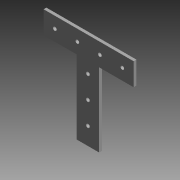
# Autodesk Inventor part: Angle attach bracket
Saved by Autodesk Inventor 2014 (Build 180170000, 170)
## iProperties
Created: 2014-01-19
Part Number: Angle attach bracket
Material: Generic
Document SubType Name: Sheet Metal
Designer: intern
Density: 1 g/cm^3
Sheet Metal Rule: Default
Appearance: Default
Author: intern
Autodesk Inventor part; units mm, degrees
ref_plane "YZ Plane" through (0, 0, 0) normal (1, 0, 0) x (0, 1, 0)
ref_plane "XZ Plane" through (0, 0, 0) normal (0, 1, 0) x (-1, 0, 0)
ref_plane "XY Plane" through (0, 0, 0) normal (0, 0, 1) x (1, 0, 0)
sketch "Sketch1" plane through (0, 0, 0) normal (0, 0, 1) x (1, 0, 0)
  line L0 (0, -83.185) -> (12.6238, -83.185)
  line L1 (12.6238, -83.185) -> (12.6238, -65.5687)
  arc A0 (12.6238, -61.4313) -> (12.6238, -65.5687) centre (12.7, -63.5) ccw
  line L2 (12.6238, -61.4313) -> (12.6238, -40.1687)
  arc A1 (12.6238, -36.0313) -> (12.6238, -40.1687) centre (12.7, -38.1) ccw
  line L3 (12.6238, -36.0313) -> (12.6238, -14.7687)
  arc A2 (12.6238, -10.6313) -> (12.6238, -14.7687) centre (12.7, -12.7) ccw
  line L4 (12.6238, -10.6313) -> (12.6238, 0)
  line L5 (0, 0) -> (12.6238, 0)
  line L6 (0, 0) -> (0, -83.185)
  line L7 (12.7762, -83.185) -> (25.4, -83.185)
  line L8 (25.4, 0) -> (25.4, -83.185)
  line L9 (12.7762, 0) -> (25.4, 0)
  line L10 (12.7762, -10.6313) -> (12.7762, 0)
  arc A3 (12.7762, -14.7687) -> (12.7762, -10.6313) centre (12.7, -12.7) ccw
  line L11 (12.7762, -36.0313) -> (12.7762, -14.7687)
  arc A4 (12.7762, -40.1687) -> (12.7762, -36.0313) centre (12.7, -38.1) ccw
  line L12 (12.7762, -61.4313) -> (12.7762, -40.1687)
  arc A5 (12.7762, -65.5687) -> (12.7762, -61.4313) centre (12.7, -63.5) ccw
  line L13 (12.7762, -83.185) -> (12.7762, -65.5687)
  line L14 (216.6911, 0) -> (216.6911, 12.6238)
  line L15 (216.6911, 12.6238) -> (206.0725, 12.6238)
  arc A6 (201.9097, 12.6238) -> (206.0725, 12.6238) centre (203.9911, 12.7) ccw
  line L16 (201.9097, 12.6238) -> (180.6725, 12.6238)
  arc A7 (176.5097, 12.6238) -> (180.6725, 12.6238) centre (178.5911, 12.7) ccw
  line L17 (176.5097, 12.6238) -> (155.2725, 12.6238)
  arc A8 (151.1097, 12.6238) -> (155.2725, 12.6238) centre (153.1911, 12.7) ccw
  line L18 (151.1097, 12.6238) -> (129.8725, 12.6238)
  arc A9 (125.7097, 12.6238) -> (129.8725, 12.6238) centre (127.7911, 12.7) ccw
  line L19 (125.7097, 12.6238) -> (104.4725, 12.6238)
  arc A10 (100.3097, 12.6238) -> (104.4725, 12.6238) centre (102.3911, 12.7) ccw
  line L20 (100.3097, 12.6238) -> (79.0725, 12.6238)
  arc A11 (74.9097, 12.6238) -> (79.0725, 12.6238) centre (76.9911, 12.7) ccw
  line L21 (74.9097, 12.6238) -> (53.6725, 12.6238)
  arc A12 (49.5097, 12.6238) -> (53.6725, 12.6238) centre (51.5911, 12.7) ccw
  line L22 (49.5097, 12.6238) -> (28.2725, 12.6238)
  arc A13 (24.1097, 12.6238) -> (28.2725, 12.6238) centre (26.1911, 12.7) ccw
  line L23 (24.1097, 12.6238) -> (2.8725, 12.6238)
  arc A14 (-1.2903, 12.6238) -> (2.8725, 12.6238) centre (0.7911, 12.7) ccw
  line L24 (-1.2903, 12.6238) -> (-22.5275, 12.6238)
  arc A15 (-26.6903, 12.6238) -> (-22.5275, 12.6238) centre (-24.6089, 12.7) ccw
  line L25 (-26.6903, 12.6238) -> (-47.9275, 12.6238)
  arc A16 (-52.0903, 12.6238) -> (-47.9275, 12.6238) centre (-50.0089, 12.7) ccw
  line L26 (-52.0903, 12.6238) -> (-73.3275, 12.6238)
  arc A17 (-77.4903, 12.6238) -> (-73.3275, 12.6238) centre (-75.4089, 12.7) ccw
  line L27 (-77.4903, 12.6238) -> (-98.7275, 12.6238)
  arc A18 (-102.8903, 12.6238) -> (-98.7275, 12.6238) centre (-100.8089, 12.7) ccw
  line L28 (-102.8903, 12.6238) -> (-124.1275, 12.6238)
  arc A19 (-128.2903, 12.6238) -> (-124.1275, 12.6238) centre (-126.2089, 12.7) ccw
  line L29 (-128.2903, 12.6238) -> (-149.5275, 12.6238)
  arc A20 (-153.6903, 12.6238) -> (-149.5275, 12.6238) centre (-151.6089, 12.7) ccw
  line L30 (-153.6903, 12.6238) -> (-174.9275, 12.6238)
  arc A21 (-179.0903, 12.6238) -> (-174.9275, 12.6238) centre (-177.0089, 12.7) ccw
  line L31 (-179.0903, 12.6238) -> (-200.3275, 12.6238)
  arc A22 (-204.4903, 12.6238) -> (-200.3275, 12.6238) centre (-202.4089, 12.7) ccw
  line L32 (-204.4903, 12.6238) -> (-225.7275, 12.6238)
  arc A23 (-229.8903, 12.6238) -> (-225.7275, 12.6238) centre (-227.8089, 12.7) ccw
  line L33 (-229.8903, 12.6238) -> (-251.1275, 12.6238)
  arc A24 (-255.2903, 12.6238) -> (-251.1275, 12.6238) centre (-253.2089, 12.7) ccw
  line L34 (-255.2903, 12.6238) -> (-276.5275, 12.6238)
  arc A25 (-280.6903, 12.6238) -> (-276.5275, 12.6238) centre (-278.6089, 12.7) ccw
  line L35 (-280.6903, 12.6238) -> (-301.9275, 12.6238)
  arc A26 (-306.0903, 12.6238) -> (-301.9275, 12.6238) centre (-304.0089, 12.7) ccw
  line L36 (-306.0903, 12.6238) -> (-327.3275, 12.6238)
  arc A27 (-331.4903, 12.6238) -> (-327.3275, 12.6238) centre (-329.4089, 12.7) ccw
  line L37 (-331.4903, 12.6238) -> (-352.7275, 12.6238)
  arc A28 (-356.8903, 12.6238) -> (-352.7275, 12.6238) centre (-354.8089, 12.7) ccw
  line L38 (-356.8903, 12.6238) -> (-378.1275, 12.6238)
  arc A29 (-382.2903, 12.6238) -> (-378.1275, 12.6238) centre (-380.2089, 12.7) ccw
  line L39 (-382.2903, 12.6238) -> (-403.5275, 12.6238)
  arc A30 (-407.6903, 12.6238) -> (-403.5275, 12.6238) centre (-405.6089, 12.7) ccw
  line L40 (-407.6903, 12.6238) -> (-418.3089, 12.6238)
  line L41 (-418.3089, 12.6238) -> (-418.3089, 0)
  line L42 (-418.3089, 0) -> (216.6911, 0)
  line L43 (216.6911, 12.7762) -> (216.6911, 25.4)
  line L44 (-418.3089, 25.4) -> (216.6911, 25.4)
  line L45 (-418.3089, 25.4) -> (-418.3089, 12.7762)
  line L46 (-418.3089, 12.7762) -> (-407.6903, 12.7762)
  arc A31 (-403.5275, 12.7762) -> (-407.6903, 12.7762) centre (-405.6089, 12.7) ccw
  line L47 (-403.5275, 12.7762) -> (-382.2903, 12.7762)
  arc A32 (-378.1275, 12.7762) -> (-382.2903, 12.7762) centre (-380.2089, 12.7) ccw
  line L48 (-378.1275, 12.7762) -> (-356.8903, 12.7762)
  arc A33 (-352.7275, 12.7762) -> (-356.8903, 12.7762) centre (-354.8089, 12.7) ccw
  line L49 (-352.7275, 12.7762) -> (-331.4903, 12.7762)
  arc A34 (-327.3275, 12.7762) -> (-331.4903, 12.7762) centre (-329.4089, 12.7) ccw
  line L50 (-327.3275, 12.7762) -> (-306.0903, 12.7762)
  arc A35 (-301.9275, 12.7762) -> (-306.0903, 12.7762) centre (-304.0089, 12.7) ccw
  line L51 (-301.9275, 12.7762) -> (-280.6903, 12.7762)
  arc A36 (-276.5275, 12.7762) -> (-280.6903, 12.7762) centre (-278.6089, 12.7) ccw
  line L52 (-276.5275, 12.7762) -> (-255.2903, 12.7762)
  arc A37 (-251.1275, 12.7762) -> (-255.2903, 12.7762) centre (-253.2089, 12.7) ccw
  line L53 (-251.1275, 12.7762) -> (-229.8903, 12.7762)
  arc A38 (-225.7275, 12.7762) -> (-229.8903, 12.7762) centre (-227.8089, 12.7) ccw
  line L54 (-225.7275, 12.7762) -> (-204.4903, 12.7762)
  arc A39 (-200.3275, 12.7762) -> (-204.4903, 12.7762) centre (-202.4089, 12.7) ccw
  line L55 (-200.3275, 12.7762) -> (-179.0903, 12.7762)
  arc A40 (-174.9275, 12.7762) -> (-179.0903, 12.7762) centre (-177.0089, 12.7) ccw
  line L56 (-174.9275, 12.7762) -> (-153.6903, 12.7762)
  arc A41 (-149.5275, 12.7762) -> (-153.6903, 12.7762) centre (-151.6089, 12.7) ccw
  line L57 (-149.5275, 12.7762) -> (-128.2903, 12.7762)
  arc A42 (-124.1275, 12.7762) -> (-128.2903, 12.7762) centre (-126.2089, 12.7) ccw
  line L58 (-124.1275, 12.7762) -> (-102.8903, 12.7762)
  arc A43 (-98.7275, 12.7762) -> (-102.8903, 12.7762) centre (-100.8089, 12.7) ccw
  line L59 (-98.7275, 12.7762) -> (-77.4903, 12.7762)
  arc A44 (-73.3275, 12.7762) -> (-77.4903, 12.7762) centre (-75.4089, 12.7) ccw
  line L60 (-73.3275, 12.7762) -> (-52.0903, 12.7762)
  arc A45 (-47.9275, 12.7762) -> (-52.0903, 12.7762) centre (-50.0089, 12.7) ccw
  line L61 (-47.9275, 12.7762) -> (-26.6903, 12.7762)
  arc A46 (-22.5275, 12.7762) -> (-26.6903, 12.7762) centre (-24.6089, 12.7) ccw
  line L62 (-22.5275, 12.7762) -> (-1.2903, 12.7762)
  arc A47 (2.8725, 12.7762) -> (-1.2903, 12.7762) centre (0.7911, 12.7) ccw
  line L63 (2.8725, 12.7762) -> (24.1097, 12.7762)
  arc A48 (28.2725, 12.7762) -> (24.1097, 12.7762) centre (26.1911, 12.7) ccw
  line L64 (28.2725, 12.7762) -> (49.5097, 12.7762)
  arc A49 (53.6725, 12.7762) -> (49.5097, 12.7762) centre (51.5911, 12.7) ccw
  line L65 (53.6725, 12.7762) -> (74.9097, 12.7762)
  arc A50 (79.0725, 12.7762) -> (74.9097, 12.7762) centre (76.9911, 12.7) ccw
  line L66 (79.0725, 12.7762) -> (100.3097, 12.7762)
  arc A51 (104.4725, 12.7762) -> (100.3097, 12.7762) centre (102.3911, 12.7) ccw
  line L67 (104.4725, 12.7762) -> (125.7097, 12.7762)
  arc A52 (129.8725, 12.7762) -> (125.7097, 12.7762) centre (127.7911, 12.7) ccw
  line L68 (129.8725, 12.7762) -> (151.1097, 12.7762)
  arc A53 (155.2725, 12.7762) -> (151.1097, 12.7762) centre (153.1911, 12.7) ccw
  line L69 (155.2725, 12.7762) -> (176.5097, 12.7762)
  arc A54 (180.6725, 12.7762) -> (176.5097, 12.7762) centre (178.5911, 12.7) ccw
  line L70 (180.6725, 12.7762) -> (201.9097, 12.7762)
  arc A55 (206.0725, 12.7762) -> (201.9097, 12.7762) centre (203.9911, 12.7) ccw
  line L71 (206.0725, 12.7762) -> (216.6911, 12.7762)
  line L72 (-37.3089, 25.4) -> (64.2911, 25.4)
  line L73 (64.2911, 25.4) -> (64.2911, 0)
  line L74 (64.2911, 0) -> (-37.3089, 0)
  line L75 (-37.3089, 0) -> (-37.3089, 25.4)
  line L76 (0, 0) -> (25.4, 0)
  line L77 (25.4, 0) -> (25.4, -83.185)
  line L78 (25.4, -83.185) -> (0, -83.185)
  line L79 (0, -83.185) -> (0, 0)
  circle A56 centre (-24.6089, 12.7) radius 2.0828
  circle A57 centre (0.7911, 12.7) radius 2.0828
  circle A58 centre (26.1911, 12.7) radius 2.0828
  circle A59 centre (51.5911, 12.6238) radius 2.0267
  circle A60 centre (12.7, -12.7) radius 2.0701
  circle A61 centre (12.7, -38.1) radius 2.0701
  circle A62 centre (12.7, -63.5) radius 2.0701
  line L80 (242.0911, -84.7725) -> (-443.7089, -84.7725)
  line L81 (242.0911, -84.7725) -> (-443.7089, -84.7725)
  line L82 (-443.7089, -86.36) -> (-443.7089, -84.7725)
  line L83 (-442.1214, -86.36) -> (-443.7089, -86.36)
  line L84 (-442.1214, -86.36) -> (240.5036, -86.36)
  line L85 (242.0911, -86.36) -> (240.5036, -86.36)
  line L86 (242.0911, -84.7725) -> (242.0911, -86.36)
  line L87 (-442.1214, -137.16) -> (-442.1214, -86.36)
  line L88 (-442.1214, -137.16) -> (240.5036, -137.16)
  line L89 (240.5036, -86.36) -> (240.5036, -137.16)
  line L90 (-442.1214, -86.36) -> (240.5036, -86.36)
  line L91 (0, -83.185) -> (25.4, -83.185)
  line L92 (0, -83.185) -> (25.4, -83.185)
  line L93 (25.4, -84.7725) -> (0, -84.7725)
  line L94 (-5.08, -83.185) -> (30.48, -83.185)
  line L95 (-5.08, -83.185) -> (30.48, -83.185)
  line L96 (-5.08, -83.185) -> (30.48, -83.185)
extrude "Plate1" add sketch "Sketch1" along normal blind 3.175 contours L6 L5 L4 A2 L3 A1 L2 A0 L1 L0 | L1 A62 L13 L78 | L42 L75 L25 A15 L24 A14 L23 A13 L22 A12 A59 L21 L73 L9 L5 | L13 A5 L12 A4 L11 A3 L10 L9 L8 L7 | L42 L10 A60 L4 | L2 A61 L12 A62 | L75 L61 A56 L25 | A60 L11 A61 L3 | L75 L44 L73 L65 A49 L64 A48 L63 A47 L62 A46 L61 | A56 L62 A57 L24 | L21 A12 A59 L22 A58 L64 A49 L65 L73 | A57 L63 A58 L23
sketch "Sketch4" plane through (25.4, -83.185, 3.175) normal (0, -1, 0) x (1, 0, 0)
  line L0 (-25.4, 0) -> (0, 0)
  line L1 (0, 0) -> (0, 85.725)
  line L2 (0, 85.725) -> (-25.4, 85.725)
  line L3 (-25.4, 85.725) -> (-25.4, 0)
  constraints: 6 end point, 1 horizontal, 1 perpendicular, 1 vertical
edge flange "Flange2" height 88.9 angle 90 thickness 3.175 bend radius 1.27 thickness toward (0, -1, 0) relief tear relief width 3.175 relief depth 1.5875 edges at (12.7, -83.185, 3.175) wall of the first edge with corners at (0, -83.185, 3.175) (25.4, -83.185, 3.175) (25.4, -83.185, 88.9) (0, -83.185, 88.9)
bend "Bend2"
corner "Corner2"
sketch "Sketch5" plane through (0, -83.185, 88.9) normal (0, 1, 0) x (1, 0, 0)
  line L0 (0, 84.455) -> (25.4, 0)
  line L1 (0, 0) -> (25.4, 84.455)
  circle A0 centre (12.7, 42.2275) radius 3.3782
  point P0 (0, 88.9)
  dimension "d29" = 6.7564
  constraints: 4 end point, 1 centre point, 1 midpoint
  measures "d29" diameter of A0
hole "Hole2" at (12.7, -83.185, 46.6725) direction (0, -1, 0) diameter 6.7564 end through all
equation "\"d35\" = Thickness"
equation "\"d19\" = BendReliefWidth"
equation "\"d20\" = BendReliefDepth"
equation "\"d21\" = MinimumRemnant"
equation "\"d22\" = BendRadius"
equation "\"d26\" = CornerReliefSize"
equation "\"d27\" = GapSize"
equation "\"d28\" = JacobiRadiusSize"
equation "\"BendRadius\" = Thickness"
equation "\"BendReliefWidth\" = Thickness"
equation "\"BendReliefDepth\" = 0.5 * Thickness"
equation "\"CornerReliefSize\" = 4 * Thickness"
equation "\"MinimumRemnant\" = 2 * Thickness"
equation "\"TransitionRadius\" = BendRadius"
equation "\"JacobiRadiusSize\" = BendRadius"
equation "\"GapSize\" = Thickness"
equation "\"d0\" = BendRadius"
equation "\"Thickness\" = 3.175"
body "Solid1"
